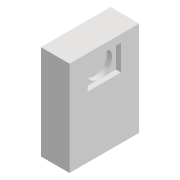
# Autodesk Inventor part: 00_huawei_p30_Objectivelensassembly
Saved by Autodesk Inventor 2022 (Build 260153000, 153)
## iProperties
Created: 2022-09-27
Part Number: 00_huawei_p30_Objectivelensassembly
Material: Generisch
Document SubType Name: Modeling
Designer: UC2
Density: 1 g/cm^3
Appearance: Vorgabe
Author: UC2
Autodesk Inventor part; units mm, degrees
ref_plane "YZ Plane" through (0, 0, 0) normal (1, 0, 0) x (0, 1, 0)
ref_plane "XZ Plane" through (0, 0, 0) normal (0, 1, 0) x (-1, 0, 0)
ref_plane "XY Plane" through (0, 0, 0) normal (0, 0, 1) x (1, 0, 0)
sketch "Skizze1" plane through (0, 0, 0) normal (1, 0, 0) x (0, 1, 0)
  line L0 (0, 0) -> (18.5, 0)
  line L1 (18.5, 0) -> (18.5, 13.6)
  line L2 (18.5, 13.6) -> (0, 13.6)
  line L3 (0, 13.6) -> (0, 0)
  dimension "d0" = 18.5
  dimension "d1" = 13.6
  constraints: 8 end point, 2 parallel, 1 horizontal, 1 perpendicular
  measures "d0" distance of L2.end L1.end
  measures "d1" distance of L1.end L0.end
extrude "Extrusion1" add sketch "Skizze1" along normal blind 5.6
sketch "Skizze2" plane through (5.6, 0, 0) normal (1, 0, 0) x (0, 0, -1)
  line L0 (0, 18.5) -> (-13.6, 18.5) projected
  line L1 (-13.6, 18.5) -> (-13.6, 0) projected
  line L2 (-13.6, 0) -> (0, 0) projected
  line L3 (0, 0) -> (0, 18.5) projected
  line L4 (-10.05, 12) -> (-3.55, 12)
  line L5 (-3.55, 12) -> (-3.55, 17)
  line L6 (-3.55, 17) -> (-10.05, 17)
  line L7 (-10.05, 17) -> (-10.05, 12)
  line L8 (-10.05, 12) -> (-3.55, 17) construction
  line L9 (-3.55, 12) -> (-10.05, 17) construction
  point P0 (-6.8, 14.5)
  dimension "d4" = 6.5
  dimension "d5" = 5
  dimension "d6" = 1.5
  constraints: 12 end point, 2 midpoint, 2 parallel, 1 horizontal, 1 perpendicular
  measures "d4" distance of L6.end L5.end
  measures "d5" distance of L5.end L4.end
  measures "d6" distance between parallel lines of L6 L0
extrude "Extrusion2" cut sketch "Skizze2" against normal blind 1 contours L7 L6 L5 L4
sketch "Skizze3" plane through (0, 0, 0) normal (0, -1, 0) x (1, 0, 0)
  line L0 (0, 13.6) -> (0, 0) projected
  line L1 (0, 0) -> (5.6, 0) projected
  line L2 (5.6, 13.6) -> (5.6, 0) projected
  line L3 (0, 13.6) -> (5.6, 13.6) projected
  circle A0 centre (2.8, 6.8) radius 2.3625
  constraints: 1 centre point
extrude "Extrusion3" cut sketch "Skizze3" against normal blind 1 contours A0
sketch "Skizze4" plane through (4.6, 0, 0) normal (1, 0, 0) x (0, 0, -1)
  line L0 (-3.55, 17) -> (-3.55, 12) projected
  line L1 (-10.05, 17) -> (-3.55, 17) projected
  line L2 (-10.05, 12) -> (-10.05, 17) projected
  line L3 (-3.55, 12) -> (-10.05, 12) projected
  circle A0 centre (-6.8, 14.5) radius 2.5
  point P0 (0, 0)
  constraints: 1 centre point
extrude "Extrusion4" cut sketch "Skizze4" against normal blind 1 contours A0
